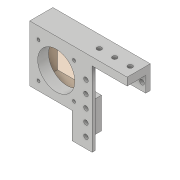
# Autodesk Inventor part: 30_CUBE_openXY_NEMA8mount
Saved by Autodesk Inventor 2019 (Build 230136000, 136)
## iProperties
Created: 2020-03-16
Part Number: 30_CUBE_openXY_NEMA8mount
Material: Generic
Document SubType Name: Modeling
Designer: diederichbenedict
Density: 1 g/cm^3
Appearance: Default
Author: diederichbenedict
Autodesk Inventor part; units mm, degrees
ref_plane "YZ Plane" through (0, 0, 0) normal (1, 0, 0) x (0, 1, 0)
ref_plane "Work Plane1" through (0, 185.6, 7) normal (0, 0, 1) x (1, 0, 0)
sketch "Sketch1" plane through (0, 185.6, 7) normal (0, 0, 1) x (1, 0, 0)
  circle A0 centre (-11.5, -11.5) radius 1 projected
  circle A1 centre (11.5, 11.5) radius 1 projected
  circle A2 centre (11.5, -11.5) radius 1 projected
  circle A3 centre (-11.5, 11.5) radius 1 projected
  circle A4 centre (0, 0) radius 11 projected
  arc A5 (-14.2, -11.025) -> (-11.025, -14.2) centre (-11.025, -11.025) ccw projected
  line L0 (-11.025, -14.2) -> (11.025, -14.2) projected
  arc A6 (11.025, -14.2) -> (14.2, -11.025) centre (11.025, -11.025) ccw projected
  line L1 (14.2, -11.025) -> (14.2, 11.025) projected
  arc A7 (14.2, 11.025) -> (11.025, 14.2) centre (11.025, 11.025) ccw projected
  line L2 (11.025, 14.2) -> (-11.025, 14.2) projected
  arc A8 (-11.025, 14.2) -> (-14.2, 11.025) centre (-11.025, 11.025) ccw projected
  line L3 (-14.2, 11.025) -> (-14.2, -11.025) projected
  line L4 (-14.2, 14.2) -> (14.2, 14.2)
  line L5 (14.2, 14.2) -> (14.2, -14.2)
  line L6 (14.2, -14.2) -> (-14.2, -14.2)
  line L7 (-14.2, -14.2) -> (-14.2, 14.2)
  circle A9 centre (-11.5, 11.5) radius 1.6
  circle A10 centre (-11.5, -11.5) radius 1.624
  circle A11 centre (11.5, -11.5) radius 1.6374
  circle A12 centre (11.5, 11.5) radius 1.6
  line L8 (14.2, -14.2) -> (10.2, -14.2)
  line L9 (10.2, -14.2) -> (10.2, -34.2)
  line L10 (10.2, -34.2) -> (14.2, -34.2)
  line L11 (14.2, -34.2) -> (14.2, -14.2)
  circle A13 centre (0, 0) radius 12
  point P0 (0, -185.6)
  dimension "d0" = 3.2
  dimension "d3" = 4
  dimension "d4" = 20
  dimension "d25" = 1
  constraints: 16 end point, 5 centre point, 4 coincident, 4 parallel, 2 horizontal, 2 perpendicular
  measures "d0" diameter of A9
  measures "d3" distance of L10.end L9.end
  measures "d4" distance of L9.end L8.end
  measures "d25" radial gap between concentric circles of A4 A13
ref_plane "Work Plane2" through (14.2, -18.2, 10) normal (0, 0, 1) x (1, 0, 0)
ref_plane "Work Plane3" through (14.2, -18.2, 8) normal (0, 0, 1) x (1, 0, 0)
extrude "Extrusion1" add sketch "Sketch1" along normal blind 5 contours L3 A8 L2 A7 L1 A6 L0 A5 | A5 L6 L7 | L7 L4 A8 | L0 L6 L11 L10 L9 | A6 L5 L6 | L4 L5 A7 | A9 | A10 | A11 | A12
sketch "Sketch2" plane through (10.2, 151.4, 7) normal (-1, 0, 0) x (0, 0, 1)
  line L0 (5, 20) -> (5, 0) projected
  line L1 (5, 0) -> (-5, 0)
  line L2 (-5, 0) -> (-5, 20)
  line L3 (-5, 20) -> (5, 20)
  line L4 (5, 20) -> (5, 0)
  point P0 (-7, -151.4)
  dimension "d30" = 10
  constraints: 8 end point, 2 parallel, 1 horizontal, 1 perpendicular
  measures "d30" distance of L2.end L3.end
extrude "Extrusion2" add sketch "Sketch2" against normal up to surface (4 mm away)
sketch "Sketch3" plane through (-14.2, 199.8, 12) normal (0, 0, 1) x (1, 0, 0)
  line L0 (28.4, 0) -> (37.4, 0)
  line L1 (37.4, 0) -> (37.4, -48.4)
  line L2 (37.4, -48.4) -> (28.4, -48.4)
  line L3 (28.4, -48.4) -> (28.4, 0)
  line L4 (34.9, -208) -> (31.9, -208) projected
  line L5 (34.9, -8) -> (34.9, -208) projected
  line L6 (31.9, -8) -> (34.9, -8) projected
  line L7 (31.9, -208) -> (31.9, -8) projected
  circle A0 centre (33.4, -25.7) radius 1.45
  circle A1 centre (33.4, -33.7) radius 1.45
  circle A2 centre (33.4, -41.7) radius 1.45
  circle A3 centre (33.4, -17.7) radius 1.45
  circle A4 centre (33.4, -25.7) radius 1.45
  circle A5 centre (33.4, -33.7) radius 1.45
  circle A6 centre (33.4, -9.7) radius 1.45
  circle A7 centre (33.4, -17.7) radius 1.45
  circle A8 centre (33.4, -25.7) radius 1.45
  circle A9 centre (14.2, -14.2) radius 12 projected
  circle A10 centre (25.7, -25.7) radius 1 projected
  circle A11 centre (2.7, -25.7) radius 1 projected
  circle A12 centre (25.7, -2.7) radius 1 projected
  circle A13 centre (2.7, -2.7) radius 1 projected
  circle A14 centre (14.2, -14.2) radius 12 projected
  line L8 (24.4, -48.4) -> (28.4, -48.4) projected
  line L9 (28.4, 0) -> (0, 0) projected
  line L10 (0, 0) -> (0, -28.4) projected
  line L11 (0, -28.4) -> (24.4, -28.4) projected
  line L12 (28.4, -48.4) -> (28.4, 0) projected
  line L13 (24.4, -28.4) -> (24.4, -48.4) projected
  point P0 (14.2, -199.8)
  dimension "d8" = 9
  dimension "d9" = 2.9
  dimension "d12" = 8
  dimension "d15" = 8
  constraints: 9 centre point, 8 end point, 2 parallel, 2 vertical, 1 horizontal, 1 perpendicular, 16 other
  measures "d8" distance of L1.end L2.end
  measures "d9" diameter of A0
  measures "d12" distance of A0.centre A1.centre
  measures "d15" distance of A0.centre A3.centre
extrude "Extrusion3" add sketch "Sketch3" along normal blind 2 contours L0 L1 L2 L5 L6 L7 L3 | L3 L8 L13 L11 L10 L9 | L7 L6 L5 L2
sketch "Sketch4" plane through (-14.2, 199.8, 7) normal (0, 1, 0) x (1, 0, 0)
  line L0 (28.4, 0) -> (0, 0) projected
  line L1 (0, 0) -> (0, -7) projected
  line L2 (28.4, 0) -> (28.4, -5) projected
  line L3 (37.4, -7) -> (0, -7) projected
  line L4 (0, -7) -> (60, -7)
  line L5 (60, -7) -> (60, 5)
  line L6 (60, 5) -> (0, 5)
  line L7 (0, 5) -> (0, -7)
  line L8 (37.4, -7) -> (0, -7) projected
  line L9 (37.4, -5) -> (37.4, -7) projected
  line L10 (37.4, -5) -> (28.4, -5) projected
  line L11 (24.4, 5) -> (28.4, 5) projected
  point P0 (14.2, 7)
  dimension "d26" = 60
  constraints: 8 end point, 2 parallel, 1 horizontal, 1 perpendicular, 1 point on line
  measures "d26" distance of L6.end L5.end
extrude "Extrusion4" add sketch "Sketch4" along normal blind 5
sketch "Sketch5" plane through (10.2, 151.4, 2) normal (-1, 0, 0) x (0, 0, 1)
  line L0 (0, 0) -> (12, 0) projected
  line L1 (12, 20) -> (12, 0) projected
  line L2 (5, 20) -> (12, 20) projected
  line L3 (0, 20) -> (5, 20) projected
  line L4 (0, 0) -> (0, 20) projected
  circle A0 centre (5, 15) radius 1.5
  circle A1 centre (5, 5) radius 1.5
  line L5 (10, 0) -> (10, 48.4) projected
  point P0 (-2, -151.4)
  dimension "d31" = 3
  dimension "d32" = 3
  dimension "d33" = 5
  dimension "d34" = 5
  dimension "d35" = 5
  dimension "d36" = 5
  constraints: 2 centre point
  measures "d31" diameter of A0
  measures "d32" diameter of A1
  measures "d33" distance from line of A1.centre L5
  measures "d34" distance from line of A0.centre L5
  measures "d35" distance from line of A1.centre L0
  measures "d36" distance from line of A0.centre L3
extrude "Extrusion5" cut sketch "Sketch5" against normal through all contours A0 | A1
sketch "Sketch6" plane through (-14.2, 171.4, 7) normal (-1, 0, 0) x (0, 0, 1)
  line L0 (0, 28.4) -> (0, 0) projected
  line L1 (0, 0) -> (7, 0) projected
  line L2 (7, 0) -> (7, 33.4) projected
  line L3 (-5, 33.4) -> (7, 33.4) projected
  line L4 (-5, 28.4) -> (-5, 33.4) projected
  line L5 (-5, 28.4) -> (0, 28.4) projected
  line L6 (7, 33.4) -> (-5, 33.4)
  line L7 (-5, 33.4) -> (-5, 0)
  line L8 (-5, 0) -> (7, 0)
  line L9 (7, 0) -> (7, 33.4)
  point P0 (-7, -171.4)
  constraints: 8 end point, 2 parallel, 1 coincident, 1 horizontal, 1 perpendicular
extrude "Extrusion6" add sketch "Sketch6" along normal blind 3
sketch "Sketch7" plane through (10.2, 171.4, 7) normal (0, -1, 0) x (1, 0, 0)
  line L0 (0, 0) -> (0, 7) projected
  line L1 (0, 7) -> (-27.4, 7) projected
  line L2 (-24.4, 0) -> (0, 0) projected
  line L3 (0, -5) -> (0, 0) projected
  line L4 (-27.4, 7) -> (0, 7)
  line L5 (0, 7) -> (0, -5)
  line L6 (0, -5) -> (-27.4, -5)
  line L7 (-27.4, -5) -> (-27.4, 7)
  line L8 (-27.4, -5) -> (-27.4, 7) projected
  line L9 (-24.4, -5) -> (-27.4, -5) projected
  line L10 (-24.4, -5) -> (-24.4, 0) projected
  point P0 (-10.2, -7)
  constraints: 8 end point, 2 parallel, 1 horizontal, 1 perpendicular
extrude "Extrusion7" add sketch "Sketch7" along normal blind 3
sketch "Sketch8" plane through (-14.2, 204.8, 7) normal (0, 1, 0) x (1, 0, 0)
  line L0 (24.4, -1.5) -> (24.4, 1.5) projected
  circle A0 centre (55, 0) radius 1.5
  line L1 (60, -7) -> (60, 5) projected
  line L2 (60, 5) -> (-3, 5) projected
  circle A1 centre (45, 0) radius 1.5
  circle A2 centre (35, 0) radius 1.5
  point P0 (14.2, 7)
  point P1 (37.4, -5)
  dimension "d43" = 3
  dimension "d44" = 5
  dimension "d45" = 5
  dimension "d48" = 10
  constraints: 3 centre point, 1 horizontal, 4 other
  measures "d43" diameter of A0
  measures "d44" distance from line of A0.centre L1
  measures "d45" vertical distance of A0.centre point (37.4, -5)
  measures "d48" distance of A0.centre A1.centre
extrude "Extrusion8" cut sketch "Sketch8" against normal through all
sketch "Sketch9" plane through (45.8, 199.8, 2) normal (0, 0, -1) x (-1, 0, 0)
  line L0 (0, 0) -> (60, 0) projected
  line L1 (60, 0) -> (60, -28.4) projected
  line L2 (63, 5) -> (63, -31.4) projected
  line L3 (0, 5) -> (63, 5) projected
  line L4 (0, 0) -> (0, 5) projected
  line L5 (0, 5) -> (31.4076, 5)
  line L6 (31.4076, 5) -> (31.4076, -10)
  line L7 (31.4076, -10) -> (0, -10)
  line L8 (0, -10) -> (0, 5)
  line L9 (0, 0) -> (60, 0) projected
  circle A0 centre (26.4076, -5) radius 1.5
  circle A1 centre (20.4076, -5) radius 1.5
  circle A2 centre (14.4076, -5) radius 1.5
  circle A3 centre (8.4076, -5) radius 1.5
  circle A4 centre (2.4076, -5) radius 1.5
  line L10 (31.6, -28.4) -> (31.6, -48.4) projected
  line L11 (35.6, -48.4) -> (31.6, -48.4) projected
  line L12 (35.6, -48.4) -> (35.6, -31.4) projected
  line L13 (63, -31.4) -> (35.6, -31.4) projected
  line L14 (60, -28.4) -> (31.6, -28.4) projected
  point P0 (45.8, -199.8)
  dimension "d55" = 10
  dimension "d56" = 3
  dimension "d57" = 5
  dimension "d58" = 5
  dimension "d61" = 6
  constraints: 8 end point, 5 centre point, 2 horizontal, 2 parallel, 1 perpendicular, 8 other
  measures "d55" distance between parallel lines of L7 L0
  measures "d56" diameter of A0
  measures "d57" distance from line of A0.centre L0
  measures "d58" distance from line of A0.centre L6
  measures "d61" distance of A0.centre A1.centre
extrude "Extrusion9" add sketch "Sketch9" along normal blind 3
body "Solid1"
